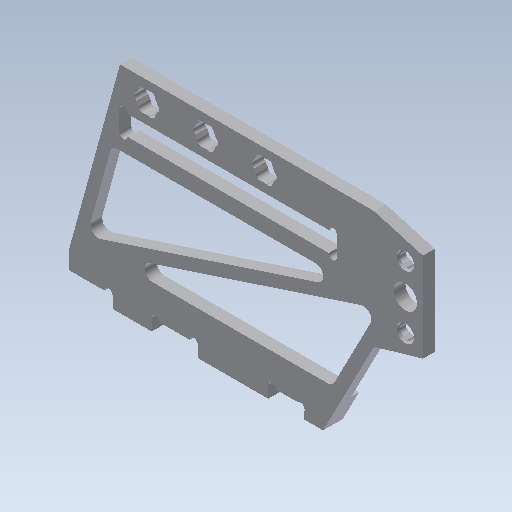
# Autodesk Inventor part: 胴体_サブフレーム_1_1
Saved by Autodesk Inventor 2020.4 (Build 244396000, 396)
## iProperties
Created: 2016-05-06
Part Number: 胴体_サブフレーム_1_1
Material: アルミニウム 2014-T4
Document SubType Name: Modeling
Designer: hiroaki
Density: 2.8 g/cm^3
Appearance: サテン
Mass: 20.7588 g
Surface Area: 71.9007 cm^2
Volume: 7.41386 cm^3
Category: 胴体
d0: 21.000 mm
d1: 1.000 mm
d2: 27.000 mm
d3: 2.700 mm
d4: 2.000 ul
d6: 27.000 mm
d7: 2.000 ul
d9: 27.000 mm
d12: 44.000 mm
d13: 32.000 mm
d14: 12.000 mm
d15: 51.500 mm
d16: 0.500 mm
d17: 72.000 mm
d18: 25.000 mm
d19: 55.000 mm
d21: 30.00 deg
d22: 25.000 mm
d23: 72.000 mm
d24: 33.500 mm
d25: 105.000 mm
d26: 5.000 mm
d27: 89.000 mm
d28: 60.000 mm
d29: 5.000 mm
d0_1: 10.100 mm
d1_1: 8.500 mm
d2_1: 2.700 mm
d3_1: 5.000 mm
d4_1: 45.00 deg
d5_1: 3.100 mm
d6_1: 5.500 mm
d7_1: 4.000 ul
d9_1: 360.00 deg
d11: 24.900 mm
d12_1: 42.000 mm
d13_1: 6.500 mm
d14_1: 2.100 mm
d15_1: 4.000 ul
d17_1: 360.00 deg
d19_1: 24.250 mm
d30: 24.250 mm
d31: 2.400 mm
d32: 4.000 ul
d34: 360.00 deg
d36: 4.000 mm
d37: 5.000 mm
d50: 2.000 mm
d51: 45.000 mm
d52: 135.00 deg
d53: 135.00 deg
d54: 59.750 mm
d60: 3.100 mm
d61: 3.000 mm
d62: 28.000 mm
d42: 2.400 mm
d44: 15.000 mm
d47: 5.000 mm
d48: 0.00 deg
d65: 2.500 mm
d69: 2.500 mm
d69_1: 51.750 mm
d72: 51.750 mm
d90: 5.000 mm
d91: 59.750 mm
d92: 1.050 mm
d93: 25.000 mm
d95: 3.000 mm
d96: 10.000 mm
d97: 43.000 mm
d98: 30.000 mm
d99: 52.000 mm
d100: 37.000 mm
d104: 55.500 mm
d105: 0.050 mm
d106: 22.000 mm
d107: 42.000 mm
d109: 5.000 mm
d110: 2.100 mm
d111: 1.050 mm
d112: 3.000 mm
d113: 51.750 mm
d114: 3.000 mm
d115: 3.100 mm
d65_1: 4.000 mm
d66_1: 6.000 mm
d68_1: 5.000 mm
d71: 6.000 mm
d72_1: 10.000 mm
d73: 5.000 mm
d74: 6.000 mm
d75: 18.000 mm
d76: 5.000 mm
d77: 2.100 mm
d78: 0.010 mm
d116: 6.000 mm
d117: 6.000 mm
d118: 10.000 mm
d119: 18.000 mm
d120: 3.000 mm
d184: 4.500 mm
d186: 16.000 mm
Author: hiroaki
Autodesk Inventor part; units mm, degrees
ref_plane "YZ Plane" through (0, 0, 0) normal (1, 0, 0) x (0, 1, 0)
ref_plane "XZ Plane" through (0, 0, 0) normal (0, 1, 0) x (-1, 0, 0)
ref_plane "XY Plane" through (0, 0, 0) normal (0, 0, 1) x (1, 0, 0)
sketch "スケッチ1" plane through (0, 0, 0) normal (0, 0, 1) x (1, 0, 0)
  line L0 (-34.75, -10) -> (23.5151, -10) construction
  arc A0 (25, -11.4849) -> (23.5151, -10) centre (24.2575, -10.7425) ccw
  line L1 (25, -11.4849) -> (25, -13)
  line L2 (25, -13) -> (30, -13)
  line L3 (23.5151, -10) -> (25, -10) construction
  line L4 (25, -10) -> (25, -11.4849) construction
  line L5 (-34.75, -10) -> (-34.75, 42)
  line L6 (-34.75, 42) -> (43, 42)
  circle A1 centre (-15, 37) radius 1.2
  circle A2 centre (15, 37) radius 1.2
  line L7 (0, 30.2) -> (0, 0) construction
  line L8 (30, -13) -> (43, 12)
  line L9 (43, 12) -> (43, 42)
  line L10 (-22.05, 32.05) -> (33.55, 32.05)
  line L11 (33.55, 32.05) -> (33.55, 26.95)
  line L12 (33.55, 26.95) -> (-22.05, 26.95)
  line L13 (-22.05, 26.95) -> (-22.05, 32.05)
  line L14 (33.5, 32) -> (-22, 32) construction
  line L15 (-22, 32) -> (-22, 27) construction
  line L16 (-22, 27) -> (33.5, 27) construction
  line L17 (33.5, 27) -> (33.5, 32) construction
  circle A3 centre (-21, 32.05) radius 1.05
  circle A4 centre (-21, 26.95) radius 1.05
  circle A5 centre (32.5, 32.05) radius 1.05
  circle A6 centre (32.5, 26.95) radius 1.05
  line L18 (-34.75, -10) -> (-25.85, -10)
  arc A7 (-23.75, -10) -> (-25.85, -10) centre (-24.8, -10) ccw
  line L19 (-23.75, -10) -> (-23.75, -13)
  line L20 (-23.75, -13) -> (-13.75, -13)
  line L21 (-13.75, -13) -> (-13.75, -10)
  arc A8 (-11.65, -10) -> (-13.75, -10) centre (-12.7, -10) ccw
  line L22 (-11.65, -10) -> (-4.1, -10)
  arc A9 (-2, -10) -> (-4.1, -10) centre (-3.05, -10) ccw
  line L23 (-2, -10) -> (-2, -13)
  line L24 (-2, -13) -> (16, -13)
  line L25 (16, -13) -> (16, -10)
  arc A10 (18.1, -10) -> (16, -10) centre (17.05, -10) ccw
  line L26 (18.1, -10) -> (23.5151, -10)
  line L27 (20.45, -6.1712) -> (23.55, -6.1712) construction
  line L28 (23.55, -6.1712) -> (23.55, -12.9737) construction
  line L29 (23.55, -12.9737) -> (20.45, -12.9737) construction
  line L30 (20.45, -12.9737) -> (20.45, -6.1712) construction
  line L31 (-31.3, -5.7897) -> (-28.2, -5.7897) construction
  line L32 (-28.2, -5.7897) -> (-28.2, -15) construction
  line L33 (-28.2, -15) -> (-31.3, -15) construction
  line L34 (-31.3, -15) -> (-31.3, -5.7897) construction
  line L35 (-29.75, -5.7897) -> (-29.75, -15) construction
  line L36 (22, -6.1712) -> (22, -12.9737) construction
  line L37 (43, 42) -> (55.5, 38.3823)
  line L38 (55.5, 38.3823) -> (55.5, 15.6177)
  line L39 (55.5, 15.6177) -> (43, 12)
  circle A11 centre (51, 35) radius 2.25
  circle A12 centre (51, 19) radius 2.25
  circle A13 centre (51, 35) radius 4.5 construction
  circle A14 centre (51, 19) radius 4.5 construction
  line L40 (51, 35) -> (51, 19) construction
  line L41 (-13.4065, 34.24) -> (-16.5935, 34.24)
  line L42 (-16.5935, 34.24) -> (-18.187, 37)
  line L43 (-18.187, 37) -> (-16.5935, 39.76)
  line L44 (-16.5935, 39.76) -> (-13.4065, 39.76)
  line L45 (-13.4065, 39.76) -> (-11.813, 37)
  line L46 (-11.813, 37) -> (-13.4065, 34.24)
  circle A15 centre (-17.137, 37) radius 1.05
  circle A16 centre (-16.0685, 35.1493) radius 1.05
  circle A17 centre (-13.9315, 35.1493) radius 1.05
  circle A18 centre (-12.863, 37) radius 1.05
  circle A19 centre (-13.9315, 38.8507) radius 1.05
  circle A20 centre (-16.0685, 38.8507) radius 1.05
  line L47 (18.187, 37) -> (16.5935, 34.24)
  line L48 (16.5935, 34.24) -> (13.4065, 34.24)
  line L49 (13.4065, 34.24) -> (11.813, 37)
  line L50 (11.813, 37) -> (13.4065, 39.76)
  line L51 (13.4065, 39.76) -> (16.5935, 39.76)
  line L52 (16.5935, 39.76) -> (18.187, 37)
  circle A21 centre (12.863, 37) radius 1.05
  circle A22 centre (13.9315, 35.1493) radius 1.05
  circle A23 centre (16.0685, 35.1493) radius 1.05
  circle A24 centre (17.137, 37) radius 1.05
  circle A25 centre (16.0685, 38.8507) radius 1.05
  circle A26 centre (13.9315, 38.8507) radius 1.05
  line L53 (1.5935, 34.24) -> (-1.5935, 34.24)
  line L54 (-1.5935, 34.24) -> (-3.187, 37)
  line L55 (-3.187, 37) -> (-1.5935, 39.76)
  line L56 (-1.5935, 39.76) -> (1.5935, 39.76)
  line L57 (1.5935, 39.76) -> (3.187, 37)
  line L58 (3.187, 37) -> (1.5935, 34.24)
  circle A27 centre (-2.137, 37) radius 1.05
  circle A28 centre (-1.0685, 35.1493) radius 1.05
  circle A29 centre (1.0685, 35.1493) radius 1.05
  circle A30 centre (2.137, 37) radius 1.05
  circle A31 centre (1.0685, 38.8507) radius 1.05
  circle A32 centre (-1.0685, 38.8507) radius 1.05
  line L59 (51, 38.1754) -> (53.75, 36.5877)
  line L60 (53.75, 36.5877) -> (53.75, 33.4123)
  line L61 (53.75, 33.4123) -> (51, 31.8246)
  line L62 (51, 31.8246) -> (48.25, 33.4123)
  line L63 (48.25, 33.4123) -> (48.25, 36.5877)
  line L64 (48.25, 36.5877) -> (51, 38.1754)
  point P0 (43, 27)
  point P1 (55.5, 27)
  point P2 (-16.5935, 34.24)
  point P3 (-13.4065, 34.24)
  point P4 (-11.813, 37)
  point P5 (-13.4065, 39.76)
  point P6 (-16.5935, 39.76)
  point P7 (16.5935, 39.76)
  point P8 (13.4065, 39.76)
  point P9 (0, 37)
  point P10 (1.5935, 39.76)
  point P11 (-1.5935, 39.76)
  dimension "d110" = 2.1
  dimension "d201" = 2.1
  dimension "d42" = 2.4
  dimension "d44" = 15
  dimension "d90" = 5
  dimension "d91" = 59.75
  dimension "d92" = 1.05
  dimension "d93" = 25
  dimension "d95" = 3
  dimension "d96" = 10
  dimension "d97" = 43
  dimension "d98" = 30
  dimension "d99" = 52
  dimension "d100" = 37
  dimension "d104" = 55.5
  dimension "d105" = 0.05
  dimension "d106" = 22
  dimension "d107" = 42
  dimension "d109" = 5
  dimension "d111" = 1.05
  dimension "d113" = 51.75
  dimension "d114" = 3
  dimension "d115" = 3.1
  dimension "d116" = 6
  dimension "d117" = 6
  dimension "d118" = 10
  dimension "d119" = 18
  dimension "d120" = 3
  dimension "d184" = 4.5
  dimension "d186" = 16
  dimension "d200" = 5.52
  dimension "d204" = 360
  dimension "d208" = 360
  dimension "d212" = 360
  dimension "d214" = 15
  dimension "d216" = 5.5
  dimension "d217" = 9
  dimension "d218" = 8
  dimension "d241" = 5
  dimension "d242" = 5
  constraints: 128 end point, 17 horizontal alignment, 11 centre point, 11 point on circle, 10 vertical, 9 horizontal, 8 parallel, 8 perpendicular, 6 equal radius, 6 midpoint, 5 coincident, 5 point on line, 4 tangent, 3 equal length, 2 vertical alignment, 182 other
  measures "d42" diameter of A1
  measures "d44" distance from line of L7 A1.centre
  measures "d90" distance of L1.end L2.end
  measures "d91" distance from line of L1 L5.start
  measures "d92" radius of A0
  measures "d93" distance between parallel lines of L1 L7
  measures "d97" distance from line of L9 point (0, 0)
  measures "d98" distance of L8.end L6.end
  measures "d100" vertical distance of point (0, 0) A1.centre
  measures "d104" distance of L14.start L14.end
  measures "d105" distance between parallel lines of L13 L15
  measures "d106" distance from line of L7.end L15
  measures "d109" distance between parallel lines of L16 L14
  measures "d111" radius of A7
  measures "d113" distance between parallel lines of L36 L35
  measures "d114" distance between parallel lines of L4 L36
  measures "d115" distance of L27.start L27.end
  measures "d116" distance between parallel lines of L35 L19
  measures "d117" distance between parallel lines of L36 L25
  measures "d118" distance of L19.end L20.end
  measures "d119" distance of L23.end L24.end
  measures "d184" diameter of A11
  measures "d186" distance of L40.start L40.end
  measures "d200" distance between parallel lines of L44 L41
  measures "d214" distance from line of A2.centre L7
  measures "d216" distance between parallel lines of L63 L60
  measures "d217" diameter of A13
  measures "d218" distance from line of L9 A11.centre
  measures "d241" distance from line of A1.centre L6
  measures "d242" distance from line of L14 A1.centre
extrude "押し出し1" add sketch "スケッチ1" along normal blind 5 contours A0 L26 A10 L25 L24 L23 A9 L22 A8 L21 L20 L19 A7 L18 L5 L6 L9 L8 L2 L1 | L9 L37 L38 L39 | L59 L60 L61 L62 L63 L64
sketch "スケッチ2" plane through (-34.75, -10, 0) normal (0, -1, 0) x (1, 0, 0)
  line L0 (0, 0) -> (0, 5)
  line L1 (8.9, 0) -> (8.9, 5) projected
  line L2 (0, 0) -> (0, 5) projected
  line L3 (59.75, 0) -> (59.75, 5) projected
  point P0 (56.75, 2.5)
  point P1 (0, 2.5)
  point P2 (5, 2.5)
  point P3 (8.9, 2.5)
  dimension "d72" = 51.75
  dimension "d112" = 3
  constraints: 3 horizontal alignment, 3 midpoint, 2 end point
  measures "d72" distance of point (56.75, 2.5) point (5, 2.5)
  measures "d112" distance from line of L3 point (56.75, 2.5)
hole "穴1" at (22, -10, 2.5) at (-29.75, -10, 2.5) direction (0, 1, 0) diameter 2.459 depth 2.5 thread size "M3x0.5" class "6H" standard "ISO Metric profile"
sketch "スケッチ9" plane through (0, 0, 0) normal (0, 0, -1) x (-1, 0, 0)
  line L0 (-18.1, -10) -> (-23.5151, -10) projected
  line L1 (19.95, 26.95) -> (-31.45, 26.95) projected
  arc A0 (-33.55, 26.95) -> (-31.45, 26.95) centre (-32.5, 26.95) ccw projected
  line L2 (-33.55, 26.95) -> (-33.55, 32.05) projected
  arc A1 (-31.45, 32.05) -> (-33.55, 32.05) centre (-32.5, 32.05) ccw projected
  line L3 (-31.45, 32.05) -> (19.95, 32.05) projected
  arc A2 (22.05, 32.05) -> (19.95, 32.05) centre (21, 32.05) ccw projected
  line L4 (22.05, 32.05) -> (22.05, 26.95) projected
  arc A3 (19.95, 26.95) -> (22.05, 26.95) centre (21, 26.95) ccw projected
  circle A4 centre (-10, 36) radius 1.2 projected
  circle A5 centre (10, 36) radius 1.2 projected
  circle A6 centre (-51, 19) radius 2.25 projected
  circle A7 centre (-51, 35) radius 2.25 projected
  line L5 (-67.988, 57.9937) -> (81.7485, 57.9937)
  line L6 (81.7485, 57.9937) -> (81.7485, -5)
  line L7 (81.7485, -5) -> (-67.988, -5)
  line L8 (-67.988, -5) -> (-67.988, 57.9937)
  point P0 (0, 0)
  dimension "d197" = 5
  constraints: 8 end point, 2 parallel, 1 horizontal, 1 perpendicular
  measures "d197" distance between parallel lines of L7 L0
extrude "押し出し5" cut sketch "スケッチ9" against normal blind 2 contours A4 | A5 | L5 L6 L7 L8
sketch "スケッチ10" plane through (0, 0, 2) normal (0, 0, -1) x (-1, 0, 0)
  line L0 (-55.5, 15.6177) -> (-55.5, 38.3823) projected
  circle A0 centre (-51, 19) radius 2.25 projected
  circle A1 centre (-51, 35) radius 2.25 projected
  line L1 (-48.25, 33.4123) -> (-51, 31.8246)
  line L2 (-51, 31.8246) -> (-53.75, 33.4123)
  line L3 (-53.75, 33.4123) -> (-53.75, 36.5877)
  line L4 (-53.75, 36.5877) -> (-51, 38.1754)
  line L5 (-51, 38.1754) -> (-48.25, 36.5877)
  line L6 (-48.25, 36.5877) -> (-48.25, 33.4123)
  line L7 (-51, 38.187) -> (-53.76, 36.5935)
  line L8 (-53.76, 36.5935) -> (-53.76, 33.4065)
  line L9 (-53.76, 33.4065) -> (-51, 31.813)
  line L10 (-51, 31.813) -> (-48.24, 33.4065)
  line L11 (-48.24, 33.4065) -> (-48.24, 36.5935)
  line L12 (-48.24, 36.5935) -> (-51, 38.187)
  circle A2 centre (-51, 37.137) radius 1.05
  circle A3 centre (-52.8507, 36.0685) radius 1.05
  circle A4 centre (-52.8507, 33.9315) radius 1.05
  circle A5 centre (-51, 32.863) radius 1.05
  circle A6 centre (-49.1493, 33.9315) radius 1.05
  circle A7 centre (-49.1493, 36.0685) radius 1.05
  line L13 (-55.5, 27) -> (-40.5359, 27) construction
  line L14 (-55.5, 15.6177) -> (-43, 12)
  line L15 (-48.25, 20.5877) -> (-51, 22.1754)
  line L16 (-51, 22.1754) -> (-53.75, 20.5877)
  line L17 (-53.75, 20.5877) -> (-53.75, 17.4123)
  line L18 (-53.75, 17.4123) -> (-51, 15.8246)
  line L19 (-51, 15.8246) -> (-48.25, 17.4123)
  line L20 (-48.25, 17.4123) -> (-48.25, 20.5877)
  line L21 (-51, 15.813) -> (-53.76, 17.4065)
  line L22 (-53.76, 17.4065) -> (-53.76, 20.5935)
  line L23 (-53.76, 20.5935) -> (-51, 22.187)
  line L24 (-51, 22.187) -> (-48.24, 20.5935)
  line L25 (-48.24, 20.5935) -> (-48.24, 17.4065)
  line L26 (-48.24, 17.4065) -> (-51, 15.813)
  circle A8 centre (-51, 16.863) radius 1.05
  circle A9 centre (-52.8507, 17.9315) radius 1.05
  circle A10 centre (-52.8507, 20.0685) radius 1.05
  circle A11 centre (-51, 21.137) radius 1.05
  circle A12 centre (-49.1493, 20.0685) radius 1.05
  circle A13 centre (-49.1493, 17.9315) radius 1.05
  point P0 (0, 0)
  point P1 (-53.76, 36.5935)
  point P2 (-53.76, 33.4065)
  point P3 (-51, 31.813)
  point P4 (-48.24, 33.4065)
  point P5 (-48.24, 36.5935)
  point P6 (-51, 19)
  point P7 (-51, 19)
  point P8 (-53.76, 17.4065)
  point P9 (-53.76, 20.5935)
  point P10 (-51, 22.187)
  point P11 (-48.24, 20.5935)
  point P12 (-48.24, 17.4065)
  dimension "d219" = 2.1
  dimension "d215" = 5.5
  dimension "d220" = 0.01
  dimension "d223" = 360
  constraints: 52 end point, 25 symmetric about line, 7 horizontal, 5 vertical alignment, 2 coincident, 1 midpoint, 1 vertical, 69 other
  measures "d215" distance between parallel lines of L6 L3
  measures "d220" distance between parallel lines of L12 L5
extrude "押し出し6" cut sketch "スケッチ10" against normal blind 2.2
sketch "スケッチ11" plane through (0, 0, 2) normal (0, 0, -1) x (-1, 0, 0)
  line L0 (-34.16, -5) -> (-43, 12) projected
  line L1 (34.75, -5) -> (-34.16, -5) projected
  line L2 (-43, 42) -> (34.75, 42) projected
  line L3 (-55.5, 15.6177) -> (-55.5, 38.3823) projected
  arc A0 (19.95, 26.95) -> (22.05, 26.95) centre (21, 26.95) ccw projected
  line L4 (-31.45, 26.95) -> (19.95, 26.95) projected
  arc A1 (-33.55, 26.95) -> (-31.45, 26.95) centre (-32.5, 26.95) ccw projected
  line L5 (-33.55, 32.05) -> (-33.55, 26.95) projected
  arc A2 (-31.45, 32.05) -> (-33.55, 32.05) centre (-32.5, 32.05) ccw projected
  line L6 (19.95, 32.05) -> (-31.45, 32.05) projected
  arc A3 (22.05, 32.05) -> (19.95, 32.05) centre (21, 32.05) ccw projected
  line L7 (22.05, 26.95) -> (22.05, 32.05) projected
  line L8 (21.2982, 44) -> (34.75, -5)
  line L9 (34.75, -5) -> (51.8772, -5)
  line L10 (51.8772, -5) -> (51.8772, 44)
  line L11 (51.8772, 44) -> (21.2982, 44)
  arc A4 (-31.5013, 32) -> (-33.5, 32.05) centre (-32.5, 32.05) ccw construction
  line L12 (-33.5, 32.05) -> (-33.5, 26.95) construction
  arc A5 (-33.5, 26.95) -> (-31.5013, 27) centre (-32.5, 26.95) ccw construction
  line L13 (-31.5013, 27) -> (20.0013, 27) construction
  arc A6 (20.0013, 27) -> (22, 26.95) centre (21, 26.95) ccw construction
  line L14 (22, 26.95) -> (22, 32.05) construction
  arc A7 (22, 32.05) -> (20.0013, 32) centre (21, 32.05) ccw construction
  line L15 (20.0013, 32) -> (-31.5013, 32) construction
  line L16 (20.0013, 32) -> (22, 32) construction
  circle A8 centre (22, 32) radius 2.5 construction
  line L17 (-45.3386, 23) -> (23.9522, 23) construction
  line L18 (23.9522, 23) -> (30.8154, -2) construction
  line L19 (30.8154, -2) -> (-32.3386, -2) construction
  line L20 (-32.3386, -2) -> (-45.3386, 23) construction
  line L21 (-45.3386, 23) -> (30.8154, -2) construction
  line L22 (-44.3487, 21.0963) -> (26.0063, -2)
  line L23 (26.0063, -2) -> (-32.3386, -2)
  line L24 (-32.3386, -2) -> (-44.3487, 21.0963)
  line L25 (-40.5295, 23) -> (23.9522, 23)
  line L26 (23.9522, 23) -> (30.3391, -0.2649)
  line L27 (30.3391, -0.2649) -> (-40.5295, 23)
  circle A9 centre (-51, 19) radius 2.25 construction
  circle A10 centre (-51, 19) radius 2.25 construction
  circle A11 centre (-51, 35) radius 2.25 construction
  circle A12 centre (-51, 35) radius 2.25 construction
  line L28 (-51, 19) -> (-51, 35) construction
  circle A13 centre (-51, 27) radius 3
  circle A14 centre (-51, 27) radius 4.5 construction
  point P0 (0, 0)
  dimension "d227" = 0.05
  dimension "d228" = 5
  dimension "d229" = 2
  dimension "d230" = 3
  dimension "d231" = 3
  dimension "d232" = 4
  dimension "d233" = 3
  dimension "d234" = 1.5
  dimension "d235" = 1.5
  constraints: 42 end point, 9 centre point, 8 point on circle, 6 horizontal, 4 collinear, 4 parallel, 4 tangent, 2 coincident, 2 vertical, 1 concentric, 1 midpoint, 1 point on line, 8 other
  measures "d227" distance between parallel lines of L6 L15
  measures "d228" diameter of A8
  measures "d229" distance between parallel lines of L11 L2
  measures "d230" distance between parallel lines of L20 L0
  measures "d231" distance between parallel lines of L1 L19
  measures "d232" distance between parallel lines of L17 L13
  measures "d233" distance between parallel lines of L8 L18
  measures "d234" distance between parallel lines of L21 L22
  measures "d235" radial gap between concentric circles of A14 A13
extrude "押し出し7" cut sketch "スケッチ11" against normal blind 5 contours L11 L10 L9 L8 | L22 L23 L24 | L25 L26 L27 | A13
fillet "フィレット4" radius 2 6 edges at (44.3487, 21.0963, 3.5) (-23.9522, 23, 3.5) (-30.3391, -0.2649, 3.5) (-26.0063, -2, 3.5) (40.5295, 23, 3.5) (32.3386, -2, 3.5)
sketch "スケッチ12" plane through (25, -13, 0) normal (-1, 0, 0) x (0, 0, 1)
  line L0 (0, 1.5151) -> (5, 1.5151) projected
  line L1 (0, 0) -> (5, 0)
  line L2 (5, 0) -> (5, 1.5151)
  line L3 (5, 1.5151) -> (0, 1.5151)
  line L4 (0, 1.5151) -> (0, 0)
  point P0 (0, 13)
  constraints: 8 end point, 2 parallel, 1 horizontal, 1 perpendicular
extrude "押し出し8" cut sketch "スケッチ12" against normal blind 0.01
equation "\"d91\" = d54"
equation "\"d72\" = d69_1"
equation "\"d54\" = 59.75"
equation "\"d69_1\" = 51.75"
